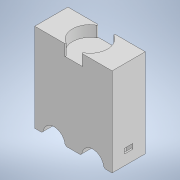
# Autodesk Inventor part: Magnet Mount
Saved by Autodesk Inventor 2022 (Build 260153000, 153)
## iProperties
Created: 2022-04-23
Part Number: Magnet Mount
Material: Generic
Document SubType Name: Modeling
Designer: Nick
Density: 1 g/cm^3
Appearance: Default
Author: Nick
Autodesk Inventor part; units mm, degrees
ref_plane "YZ Plane" through (0, 0, 0) normal (1, 0, 0) x (0, 1, 0)
ref_plane "XZ Plane" through (0, 0, 0) normal (0, 1, 0) x (-1, 0, 0)
ref_plane "XY Plane" through (0, 0, 0) normal (0, 0, 1) x (1, 0, 0)
sketch "Sketch1" plane through (0, 0, 0) normal (0, 0, 1) x (1, 0, 0)
  line L0 (0, 0) -> (28, 0)
  line L1 (28, 0) -> (28, 32)
  line L2 (28, 32) -> (0, 32)
  line L3 (0, 32) -> (0, 0)
  circle A0 centre (7, 0) radius 4
  circle A1 centre (21, 0) radius 4
  point P0 (3, 0)
  point P1 (11, 0)
  point P2 (17, 0)
  point P3 (25, 0)
  dimension "d0" = 28
  dimension "d1" = 32
  dimension "d2" = 8
  dimension "d3" = 8
  dimension "d4" = 14
  dimension "d5" = 7
  dimension "d6" = 7
  constraints: 8 end point, 2 centre point, 2 parallel, 2 point on line, 1 horizontal, 1 perpendicular
  measures "d0" distance of L2.end L1.end
  measures "d1" distance of L1.end L0.end
  measures "d2" diameter of A0
  measures "d3" diameter of A1
  measures "d4" distance of A0.centre A1.centre
  measures "d5" distance of L0.end A1.centre
  measures "d6" distance from line of L3 A0.centre
extrude "Extrusion1" add sketch "Sketch1" along normal blind 12 contours A1 L0 A0 L3 L2 L1
chamfer "Chamfer1" distance 0.5 angle 45 4 edges at (3, 0, 6) (11, 0, 6) (17, 0, 6) (25, 0, 6)
sketch "Sketch2" plane through (0, 32, 0) normal (0, 1, 0) x (1, 0, 0)
  circle A0 centre (14, -6) radius 6.35
  line L0 (28, 0) -> (0, 0) projected
  line L1 (28, 0) -> (28, -12) projected
  point P0 (14, 0)
  point P1 (28, -6)
  point P2 (16.0791, 0)
  point P3 (11.9209, 0)
  dimension "d12" = 12.7
  constraints: 2 midpoint, 1 centre point, 1 horizontal alignment, 1 vertical alignment
  measures "d12" diameter of A0
extrude "Extrusion2" cut sketch "Sketch2" against normal blind 4 contours A0 L0 picked at (13.6383, -8.0675)
fillet "Fillet1" radius 0.25 4 edges at (11.9209, 30, 0) (16.0791, 30, 0) (16.0791, 30, 12) (11.9209, 30, 12)
sketch "Sketch3" plane through (28, 0, 0) normal (1, 0, 0) x (0, 0, -1)
  line L0 (-7.5, 5.5) -> (-4.5, 5.5)
  line L1 (-4.5, 5.5) -> (-4.5, 4)
  line L2 (-4.5, 4) -> (-7.5, 4)
  line L3 (-7.5, 4) -> (-7.5, 5.5)
  line L4 (0, 0) -> (-12, 0) projected
  point P0 (-6, 4)
  point P1 (-6, 0)
  dimension "d16" = 3
  dimension "d17" = 1.5
  dimension "d18" = 4
  constraints: 8 end point, 2 midpoint, 2 parallel, 1 horizontal, 1 perpendicular, 1 vertical alignment
  measures "d16" distance of L1.end L2.end
  measures "d17" distance of L0.end L1.end
  measures "d18" distance between parallel lines of L4 L2
ref_plane "Work Plane1" through (0, 0, 6) normal (0, 0, 1) x (1, 0, 0)
sketch "Sketch4" plane through (0, 0, 6) normal (0, 0, 1) x (1, 0, 0)
  arc A0 (24.9688, 0.499) -> (17.0313, 0.499) centre (21, 0) ccw projected
  line L0 (24.9688, 0.499) -> (28, 0.499)
  line L1 (28, 0) -> (28, 32) projected
  line L2 (25.5, 0) -> (28, 0) projected
  line L3 (26.4844, 0) -> (26.4844, 3.2344)
  line L4 (28, 5.5) -> (28, 4) projected
  arc A1 (28, 4.75) -> (26.4844, 3.2344) centre (28, 3.2344) ccw
  line L5 (28, 4.75) -> (26.3546, 4.75) construction
  point P0 (0, 0)
  point P1 (26.4844, 0.499)
  constraints: 6 end point, 3 point on line, 2 midpoint, 2 perpendicular, 2 point on circle, 2 tangent, 1 centre point, 1 horizontal
sweep "Sweep1" cut profiles "Sketch3" path "Sketch4" path curves A1 L3
fillet "Fillet2" radius 0.25 1 edges at (28, 4, 6)
ref_plane "Work Plane2" through (14, 0, 0) normal (1, 0, 0) x (0, 0, -1)
mirror "Mirror1" about plane through (14, 0, 0) normal (1, 0, 0) of "Sweep1", "Fillet2"
equation "\"d1\" = MotorHeight"
equation "\"d5\" = d6"
equation "\"MotorHeight\" = MotorHeightBase"
equation "\"MotorHeightBase\" = 32"
body "Solid1"
